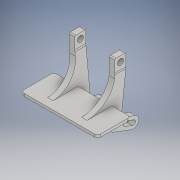
# Autodesk Inventor part: AUX_batterry_mount
Saved by Autodesk Inventor 2019 (Build 230136000, 136)
## iProperties
Created: 2019-11-16
Part Number: AUX_batterry_mount
Material: Generic
Document SubType Name: Modeling
Designer: steve
Density: 1 g/cm^3
Appearance: Default
Author: steve
Autodesk Inventor part; units mm, degrees
ref_plane "YZ Plane" through (0, 0, 0) normal (1, 0, 0) x (0, 1, 0)
ref_plane "XZ Plane" through (0, 0, 0) normal (0, 1, 0) x (-1, 0, 0)
ref_plane "XY Plane" through (0, 0, 0) normal (0, 0, 1) x (1, 0, 0)
sketch "Sketch3" plane through (0, 0, 0) normal (0, 0, 1) x (1, 0, 0)
  line L0 (41.55, 0) -> (41.55, -24)
  line L1 (41.55, -24) -> (33, -107)
  line L2 (33, -107) -> (23, -107)
  line L3 (23, -107) -> (31.55, -24)
  line L4 (31.55, -24) -> (31.55, 0)
  line L5 (31.55, 0) -> (41.55, 0)
  line L6 (-8.31, 0) -> (49.86, 0) projected
  point P0 (0, 0)
  dimension "barWidth" = 10
  dimension "d33" = 24
  dimension "d37" = 23
  dimension "d38" = 41.55
  dimension "d39" = 107
  constraints: 12 end point, 2 parallel, 2 perpendicular, 1 horizontal, 1 point on line, 1 vertical
  measures "barWidth" distance between parallel lines of L0 L4
  measures "d33" distance of L0.start L0.end
  measures "d37" horizontal distance of point (0, 0) L2.end
  measures "d38" distance of L0.start point (0, 0)
  measures "d39" distance between parallel lines of L5 L2
extrude "Extrusion2" add sketch "Sketch3" along normal blind 20
ref_plane "Work Plane1" through (23, -107, 0) normal (1, 0, 0) x (0, 0, 1)
sketch "Sketch4" plane through (23, -107, 0) normal (1, 0, 0) x (0, 0, 1)
  arc A0 (-18.4663, 28.3548) -> (-25.5337, 9.6452) centre (-22, 19) ccw
  line L0 (-25.5337, 9.6452) -> (0, 0)
  line L1 (20, 0) -> (0, 0)
  line L2 (0, 0) -> (20, 0) projected
  line L3 (-22, 19) -> (-7.9678, 13.6994) construction
  line L4 (-23.4135, 15.2581) -> (-9.3812, 9.9575)
  line L5 (-6.5543, 17.4414) -> (-20.5865, 22.7419)
  arc A1 (-20.5865, 22.7419) -> (-23.4135, 15.2581) centre (-22, 19) ccw
  arc A2 (-9.3812, 9.9575) -> (-6.5543, 17.4414) centre (-7.9678, 13.6994) ccw
  line L6 (20, 0) -> (20, 13.8245)
  line L7 (20, 13.8245) -> (-18.4663, 28.3548)
  line L8 (20, 0) -> (20, -83) projected
  line L9 (0, -83) -> (0, 0) projected
  point P0 (0, -107)
  point P1 (-14.9839, 16.3497)
  dimension "d23" = 15
  dimension "d40" = 8
  dimension "d41" = 20
  dimension "d42" = 20
  dimension "d43" = 22
  constraints: 16 end point, 6 point on circle, 6 tangent, 3 centre point, 3 parallel, 1 midpoint, 1 vertical
  measures "d23" distance of L3.start L3.end
  measures "d40" distance between parallel lines of L4 L5
  measures "d41" distance between parallel lines of L0 L7
  measures "d42" distance between parallel lines of L8 L9
  measures "d43" distance from line of L9 L3.start
extrude "Extrusion4" add sketch "Sketch4" along normal blind 10
fillet "Fillet1" radius 2 2 edges at (36.55, 0, 20) (36.55, 0, 0)
sketch "Sketch5" plane through (41.55, -24, 20) normal (1, 0, 0) x (0, 0, -1)
  circle A0 centre (10, 14) radius 5.5
  line L0 (20, 22) -> (20, 0) projected
  line L1 (0, 0) -> (0, 22) projected
  line L2 (18, 24) -> (2, 24) projected
  point P0 (20, 24)
  dimension "d29" = 11
  dimension "d30" = 20
  dimension "d31" = 10
  dimension "d32" = 10
  constraints: 1 centre point
  measures "d29" diameter of A0
  measures "d30" distance between parallel lines of L0 L1
  measures "d31" distance from line of L1 A0.centre
  measures "d32" distance from line of L2 A0.centre
extrude "Extrusion5" cut sketch "Sketch5" against normal up to next
fillet "Fillet2" radius 8.25 1 edges at (28, -120.8245, 20)
fillet "Fillet3" radius 32.5 2 edges at (41.55, -24, 10) (31.55, -24, 10)
mirror "Mirror1" about plane through (0, 0, 0) normal (1, 0, 0)
sketch "Sketch6" plane through (0, 0, 20) normal (0, 0, 1) x (1, 0, 0)
  line L0 (70, -82.2581) -> (-70, -82.2581)
  line L1 (-70, -82.2581) -> (-70, -77.2581)
  line L2 (-70, -77.2581) -> (70, -77.2581)
  line L3 (70, -77.2581) -> (70, -82.2581)
  line L4 (33, -122.2581) -> (33, -130) projected
  point P0 (0, 0)
  point P1 (33, -129.7419)
  dimension "d46" = 140
  dimension "d47" = 5
  dimension "d48" = 70
  dimension "d57" = 40
  constraints: 8 end point, 2 parallel, 1 horizontal, 1 perpendicular
  measures "d46" distance of L0.start L0.end
  measures "d47" distance between parallel lines of L0 L2
  measures "d48" distance from line of point (0, 0) L1
  measures "d57" distance from line of L0 L4.start
extrude "Extrusion6" add sketch "Sketch6" along normal blind 60
fillet "Fillet4" radius 45.5 2 edges at (31.0638, -77.2581, 20) (-31.0638, -77.2581, 20)
fillet "Fillet5" radius 6 4 edges at (70, -79.7581, 20) (70, -79.7581, 80) (-70, -79.7581, 80) (-70, -79.7581, 20)
equation "\"d41\" = d42"
equation "\"d24\" = barWidth"
equation "\"d31\" = 0.5 * d30"
equation "\"d27\" = barWidth"
equation "\"d48\" = 0.5 * d46"
body "Solid2"
